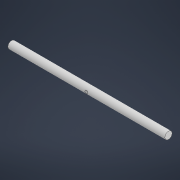
# Autodesk Inventor part: Eixo_dianteiro
Saved by Autodesk Inventor 2022 (Build 260153000, 153)
## iProperties
Created: 2022-06-10
Part Number: Eixo_dianteiro
Material: Generic
Document SubType Name: Modeling
Designer: Gugarauj07
Density: 1 g/cm^3
Appearance: Default
Author: Gugarauj07
Autodesk Inventor part; units mm, degrees
ref_plane "YZ Plane" through (0, 0, 0) normal (1, 0, 0) x (0, 1, 0)
ref_plane "XZ Plane" through (0, 0, 0) normal (0, 1, 0) x (-1, 0, 0)
ref_plane "XY Plane" through (0, 0, 0) normal (0, 0, 1) x (1, 0, 0)
sketch "Sketch1" plane through (0, 0, 0) normal (0, 0, 1) x (1, 0, 0)
  line L0 (-275, 12.7) -> (275, 12.7)
  line L1 (275, 12.7) -> (275, -12.7)
  line L2 (275, -12.7) -> (-275, -12.7)
  line L3 (-275, -12.7) -> (-275, 12.7)
  line L4 (-275, 12.7) -> (275, -12.7) construction
  line L5 (275, 12.7) -> (-275, -12.7) construction
  circle A0 centre (0, 0) radius 5
  dimension "d0" = 550
  dimension "d1" = 25.4
  dimension "d2" = 10
  constraints: 12 end point, 2 midpoint, 2 parallel, 1 centre point, 1 coincident, 1 horizontal, 1 perpendicular
  measures "d0" distance of L1.end L2.end
  measures "d1" distance of L0.end L1.end
  measures "d2" diameter of A0
extrude "Extrusion1" add sketch "Sketch1" along normal blind 25.4
fillet "Fillet1" radius 12.7 4 edges at (0, 12.7, 0) (0, -12.7, 0) (0, 12.7, 25.4) (0, -12.7, 25.4)
body "Solid1"
